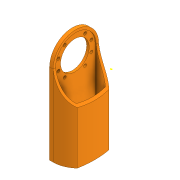
# Autodesk Inventor part: Axis 2 Arm
Saved by Autodesk Inventor 2020 (Build 240168000, 168)
## iProperties
Created: 2021-06-30
Part Number: Axis 2 Arm
Material: Generic
Document SubType Name: Modeling
Designer: Coy
Density: 1 g/cm^3
Appearance: Orange
Author: Coy
Autodesk Inventor part; units mm, degrees
ref_plane "YZ Plane" through (0, 0, 0) normal (1, 0, 0) x (0, 1, 0)
ref_plane "XZ Plane" through (0, 0, 0) normal (0, 1, 0) x (-1, 0, 0)
ref_plane "XY Plane" through (0, 0, 0) normal (0, 0, 1) x (1, 0, 0)
sketch "Sketch1" plane through (0, 0, 0) normal (1, 0, 0) x (0, 1, 0)
  line L0 (150, 47.6174) -> (150, 47.7254)
  circle A0 centre (88.3156, 92.8725) radius 3
  circle A1 centre (31.6844, 92.8725) radius 3
  circle A2 centre (49.1844, 105.587) radius 3
  circle A3 centre (31.6844, 51.7275) radius 3
  circle A4 centre (70.8156, 39.013) radius 3
  circle A5 centre (88.3156, 51.7275) radius 3
  circle A6 centre (70.8156, 105.587) radius 3
  circle A7 centre (49.1844, 39.013) radius 3
  circle A8 centre (59.99, 72.3) radius 30 construction
  arc A9 (59.99, 32.3) -> (59.99, 112.3) centre (59.99, 72.3) ccw construction
  line L1 (-103.2, -308.2363) -> (-103.2, 417.5733)
  line L2 (-103.2, 112.3) -> (59.99, 112.3) construction
  line L3 (-103.2, 32.3) -> (59.99, 32.3) construction
  circle A10 centre (59.99, 72.3) radius 29
  line L4 (-103.2, 113.3) -> (59.99, 113.3)
  arc A11 (59.99, 31.3) -> (59.99, 113.3) centre (59.99, 72.3) ccw
  line L5 (59.99, 31.3) -> (-103.2, 31.3)
  line L6 (-103.2, 118.3) -> (59.99, 118.3)
  arc A12 (59.99, 26.3) -> (59.99, 118.3) centre (59.99, 72.3) ccw
  line L7 (59.99, 26.3) -> (-103.2, 26.3)
  point P0 (0, 0)
  point P1 (233, 72.3)
  point P2 (10, 134.109)
  point P3 (10, 10.5626)
  point P4 (-223, 72.3)
  point P5 (102.0387, 41.8672)
  point P6 (101.8384, 104.9787)
  point P7 (44.6465, 123.1195)
  point P8 (45.2345, 22.5467)
  dimension "d3" = 60
  dimension "d5" = 6
  dimension "d6" = 6
  dimension "d7" = 6
  dimension "d8" = 6
  dimension "d9" = 6
  dimension "d10" = 6
  dimension "d11" = 6
  dimension "d12" = 6
  dimension "d13" = 123.19
  dimension "d16" = 1
  dimension "d17" = 1
  dimension "d18" = 5
  constraints: 16 end point, 13 centre point, 6 point on circle, 2 perpendicular, 2 point on line, 2 tangent, 1 coincident, 1 vertical, 4 other
  measures "d3" diameter of A8
  measures "d5" diameter of A1
  measures "d6" diameter of A2
  measures "d7" diameter of A6
  measures "d8" diameter of A0
  measures "d9" diameter of A5
  measures "d10" diameter of A4
  measures "d11" diameter of A7
  measures "d12" diameter of A3
  measures "d13" distance edge to line of A9 L1
  measures "d16" radial gap between concentric circles of A8 A10
  measures "d17" radial gap between concentric circles of A9 A11
  measures "d18" radial gap between concentric circles of A11 A12
extrude "Extrusion1" add sketch "Sketch1" along normal blind 5
sketch "Sketch2" plane through (5, 0, 0) normal (1, 0, 0) x (0, 0, -1)
  point P0 (0, 0)
sketch "Sketch3" plane through (5, 0, 0) normal (1, 0, 0) x (0, 0, -1)
  arc A0 (-26.3, 59.99) -> (-118.3, 59.99) centre (-72.3, 59.99) ccw projected
  line L0 (-118.3, 59.99) -> (-118.3, -103.2) projected
  line L1 (-26.3, -103.2) -> (-26.3, 59.99) projected
  line L2 (-113.3, -103.2) -> (-113.3, 59.99)
  arc A1 (-31.3, 59.99) -> (-113.3, 59.99) centre (-72.3, 59.99) ccw
  line L3 (-31.3, 59.99) -> (-31.3, -103.2)
  line L4 (-118.3, -103.2) -> (-26.3, -103.2) projected
  point P0 (0, 0)
  dimension "d19" = 5
  constraints: 4 end point, 2 point on circle, 1 centre point, 2 other
  measures "d19" radial gap between concentric circles of A0 A1
extrude "Extrusion2" add sketch "Sketch3" along normal blind 2 contours L1 L4 L3 A1 L2 L0 A0
sketch "Sketch4" plane through (7, 0, 0) normal (1, 0, 0) x (0, 0, -1)
  point P0 (0, 0)
sketch "Sketch5" plane through (0, -103.2, 26.3) normal (0, -1, 0) x (1, 0, 0)
  line L0 (7, 92) -> (7, 87) projected
  line L1 (7, 5) -> (7, 0) projected
  line L2 (45, -28.0637) -> (45, 114.6404) construction
  line L3 (0, 92) -> (0, 0) construction
  line L4 (0, 0) -> (7, 0) projected
  line L5 (0, 0) -> (7, 0) projected
  arc A0 (7, 0) -> (42, 14) centre (7, 50.75) ccw
  line L6 (7, 0) -> (7, 92) projected
  line L7 (42, 14) -> (42, 78) construction
  arc A1 (42, 14) -> (42, 78) centre (-127.1667, 46) ccw
  line L8 (7, 46) -> (75.2721, 46) construction
  arc A2 (42, 78) -> (7, 92) centre (7, 41.25) ccw
  line L9 (0, 92) -> (7, 92) construction
  arc A3 (37.385, 75.4526) -> (7, 87) centre (7, 41.25) ccw
  arc A4 (37.385, 16.5474) -> (37.385, 75.4526) centre (-127.1667, 46) ccw
  arc A5 (7, 5) -> (37.385, 16.5474) centre (7, 50.75) ccw
  point P0 (0, -26.3)
  dimension "d22" = 45
  dimension "d23" = 32
  dimension "d24" = 64
  dimension "d25" = 3
  dimension "d26" = 5
  constraints: 12 point on circle, 6 centre point, 6 end point, 3 tangent, 2 vertical, 1 horizontal, 1 midpoint, 2 other
  measures "d22" distance between parallel lines of L3 L2
  measures "d23" vertical distance of L7.start L8.start
  measures "d24" distance of L7.start L7.end
  measures "d25" distance between parallel lines of L2 L7
  measures "d26" radial gap between concentric circles of A1 A4
extrude "Extrusion3" add sketch "Sketch5" against normal blind 163 contours A2 A1 A0 L1 A5 A4 A3 L0
sketch "Sketch6" plane through (0, -103.2, 118.3) normal (0, 0, 1) x (1, 0, 0)
  line L0 (5, 192.19) -> (5, 134.19) construction
  line L1 (0, 192.19) -> (0, 134.19) construction
  line L2 (-87.708, 104.19) -> (149.8577, 104.19) construction
  line L3 (7, 163) -> (7, 0) projected
  line L4 (45, 0) -> (45, 163) projected
  arc A0 (7, 163) -> (45, 104.19) centre (87.6118, 173.4054) ccw
  line L5 (42, 163) -> (7, 163) projected
  line L6 (45, 163) -> (42, 163) projected
  line L7 (45, 0) -> (45, 163) projected
  point P0 (0, 103.2)
  dimension "d29" = 30
  constraints: 2 end point, 2 point on circle, 2 point on line, 1 centre point, 1 horizontal
  measures "d29" distance from line of L0.end L2
extrude "Extrusion4" cut sketch "Sketch6" against normal blind 163
sketch "Sketch8" plane through (0, 0, 0) normal (-1, 0, 0) x (0, 0, 1)
  line L0 (-51.3471, -60.7) -> (172.6646, -60.7) construction
  line L1 (118.3, -103.2) -> (26.3, -103.2) construction
  line L2 (113.3, -103.2) -> (31.3, -103.2) construction
  line L3 (72.3, -103.2) -> (72.3, -13.889) construction
  circle A0 centre (87.3, -60.7) radius 3.45
  circle A1 centre (57.3, -60.7) radius 3.45
  point P0 (0, 0)
  dimension "d32" = 42.5
  dimension "d33" = 15
  dimension "d34" = 15
  dimension "d35" = 6.9
  dimension "d36" = 6.9
  constraints: 4 end point, 2 centre point, 2 coincident, 2 point on line, 1 horizontal, 1 midpoint, 1 vertical
  measures "d32" distance between parallel lines of L1 L0
  measures "d33" distance from line of point (57.3, -60.7) L3
  measures "d34" distance from line of L3 point (87.3, -60.7)
  measures "d35" diameter of A0
  measures "d36" diameter of A1
extrude "Extrusion5" cut sketch "Sketch8" against normal blind 8
sketch "Sketch9" plane through (5, 0, 0) normal (1, 0, 0) x (0, 0, -1)
  circle A0 centre (-57.3, -60.7) radius 3.45 projected
  circle A1 centre (-87.3, -60.7) radius 3.45 projected
  circle A2 centre (-57.3, -60.7) radius 3.45 projected
  circle A3 centre (-57.3, -60.7) radius 6
  circle A4 centre (-87.3, -60.7) radius 3.45 projected
  circle A5 centre (-87.3, -60.7) radius 6
  point P0 (0, 0)
  dimension "d39" = 12
  dimension "d40" = 12
  constraints: 2 centre point, 2 coincident
  measures "d39" diameter of A3
  measures "d40" diameter of A5
extrude "Extrusion6" add sketch "Sketch9" along normal blind 3
sketch "Sketch10" plane through (8, -60.7, 57.3) normal (1, 0, 0) x (0, 0, -1)
  circle A0 centre (0, 0) radius 6 projected
  circle A1 centre (-30, 0) radius 6 projected
  point P0 (57.3, 60.7)
extrude "Extrusion7" add sketch "Sketch10" along normal blind 3
equation "\"d24\" = 2 * d23"
equation "\"d36\" = d35"
body "Solid1"
